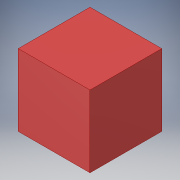
# Autodesk Inventor part: Cube
Saved by Autodesk Inventor 2019.3 (Build 233278000, 278)
## iProperties
Created: 2019-03-04
Part Number: Cube
Material: Plastique ABS
Document SubType Name: Modeling
Designer: Houba Guillaume
Mass: 67.84 g
Surface Area: 96 cm^2
Volume: 64 cm^3
Density: 1.06 g/cm^3
Appearance: Lisse - Rouge
Author: Houba Guillaume
## iProperties of the stored document Cube_Impression 3D.ipt
Created: 2019-03-04
Part Number: Cube_Impression 3D
Material: Générique
Document SubType Name: Modeling
Designer: Houba Guillaume
Mass: 64 g
Surface Area: 96 cm^2
Volume: 64 cm^3
Density: 1 g/cm^3
Appearance: Par défaut
Author: Houba Guillaume
Autodesk Inventor part; units mm, degrees
ref_plane "YZ Plane" through (0, 0, 0) normal (1, 0, 0) x (0, 1, 0)
ref_plane "XZ Plane" through (0, 0, 0) normal (0, 1, 0) x (-1, 0, 0)
ref_plane "XY Plane" through (0, 0, 0) normal (0, 0, 1) x (1, 0, 0)
sketch "Esquisse1" plane through (0, 0, 0) normal (0, 1, 0) x (-1, 0, 0)
  line L0 (-12.7, 27.3) -> (27.3, 27.3)
  line L1 (27.3, 27.3) -> (27.3, -12.7)
  line L2 (27.3, -12.7) -> (-12.7, -12.7)
  line L3 (-12.7, -12.7) -> (-12.7, 27.3)
  line L4 (-23.1177, 7.3) -> (27.6823, 7.3) construction
  line L5 (7.3, 29.243) -> (7.3, -21.557) construction
  dimension "d0" = 20
  dimension "d1" = 20
  constraints: 12 end point, 3 perpendicular, 2 parallel, 1 horizontal, 2 other
  measures "d0" distance between parallel lines of L3 L5
  measures "d1" distance between parallel lines of L4 L2
extrude "Bloc1" add sketch "Esquisse1" along normal blind 40
equation "\"d0\" = 0.5 * dd0"
equation "\"d1\" = 0.5 * dd0"
equation "\"d2\" = dd0"
equation "\"dd0\" = 40"
